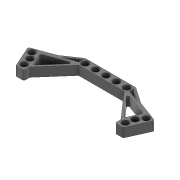
# Autodesk Inventor part: 2020-04-02-10-10501-LED_Splitter_Transparent
Saved by Autodesk Inventor 2020 (Build 240168000, 168)
## iProperties
Created: 2020-11-03
Part Number: 2020-04-02-10-10501-LED_Splitter_Transparent
Material: ABS Plastic
Document SubType Name: Modeling
Designer: eunde
Density: 1.06 g/cm^3
Appearance: Smooth - Black
Author: eunde
Autodesk Inventor part; units mm, degrees
ref_plane "YZ Plane" through (0, 0, 0) normal (1, 0, 0) x (0, 1, 0)
ref_plane "XZ Plane" through (0, 0, 0) normal (0, 1, 0) x (-1, 0, 0)
ref_plane "XY Plane" through (0, 0, 0) normal (0, 0, 1) x (1, 0, 0)
sketch "Sketch1" plane through (0, 0, 0) normal (0, 1, 0) x (-1, 0, 0)
  circle A0 centre (39, -6.055) radius 2.6
  circle A1 centre (40.5, -12.055) radius 2.6
  circle A2 centre (44, -17.055) radius 2.6
  line L0 (48.784, -18.8092) -> (41.3, -2)
  line L1 (0, 0) -> (60.8895, 0) construction
  line L2 (41.3, -2) -> (35.1, -2)
  circle A3 centre (16, -30.05) radius 2.6
  circle A4 centre (8, -30.05) radius 2.6
  arc A5 (0, -32.65) -> (0, -27.45) centre (0, -30.05) ccw
  line L3 (0, -33.55) -> (0, -32.65)
  line L4 (0, -27.45) -> (0, -26.55)
  line L5 (35.1, -2) -> (35.1, -6.5)
  line L6 (35.1, -8.7741) -> (39.6892, -19.0815)
  line L7 (0, -33.55) -> (19.5, -33.55)
  line L8 (19.5, -31.7318) -> (19.5, -28.6602)
  line L9 (19.5, -33.55) -> (31.902, -25.0543)
  line L10 (19.5, -31.7318) -> (29.2478, -25.0543)
  line L11 (17.5043, -26.55) -> (35.1, -6.5)
  line L12 (19.5, -26.55) -> (35.1, -8.7741)
  line L13 (19.5, -28.6602) -> (29.2478, -25.0543)
  line L14 (0, -26.55) -> (17.5043, -26.55)
  line L15 (39.6892, -19.0815) -> (19.5, -26.55)
  line L16 (48.784, -18.8092) -> (31.902, -25.0543)
  dimension "d0" = 5.2
  dimension "d1" = 1.5
  dimension "d3" = 3.5
  dimension "d5" = 6
  dimension "d6" = 5
  dimension "d12" = 39
  dimension "d14" = 114
  dimension "d15" = 18.4
  dimension "d16" = 6.055
  dimension "d17" = 6.2
  dimension "d19" = 30.05
  dimension "d21" = 8
  dimension "d22" = 5.2
  dimension "d26" = 3.9
  dimension "d29" = 19.5
  dimension "d31" = 18
  dimension "d35" = 1.5
  dimension "d37" = 1.5
  dimension "d40" = 3.5
  dimension "d41" = 3.5
  dimension "d44" = 4.5
  dimension "d45" = 0
  dimension "d46" = 8
  dimension "d48" = 2.9
  dimension "d49" = 2
  dimension "d51" = 0
  constraints: 34 end point, 7 vertical alignment, 6 centre point, 4 equal radius, 4 horizontal alignment, 3 horizontal, 3 vertical, 2 perpendicular, 2 point on circle
  measures "d0" diameter of A2
  measures "d1" horizontal distance of A0.centre A1.centre
  measures "d3" horizontal distance of A1.centre A2.centre
  measures "d5" vertical distance of A1.centre A0.centre
  measures "d6" vertical distance of A2.centre A1.centre
  measures "d12" horizontal distance of L1.start A0.centre
  measures "d14" angle of L1 L0
  measures "d15" distance of L0.start L0.end
  measures "d16" distance from line of L1 A0.centre
  measures "d17" distance of L0.end L2.end
  measures "d19" distance from line of L1 A3.centre
  measures "d21" distance of A3.centre A4.centre
  measures "d22" diameter of A5
  measures "d26" horizontal distance of L2.end A0.centre
  measures "d29" distance of L3.start L7.end
  measures "d31" distance of L9.end L0.start
  measures "d35" distance between parallel lines of L9 L10
  measures "d37" distance between parallel lines of L12 L11
  measures "d40" vertical distance of L3.start A4.centre
  measures "d41" distance of A5.centre L4.end
  measures "d44" distance of L2.end L5.end
  measures "d45" angle of L0 L6
  measures "d46" distance of A5.centre A4.centre
  measures "d48" distance between parallel lines of L16 L15
  measures "d49" distance between parallel lines of L1 L2
  measures "d51" angle of L13 L15
extrude "Extrusion1" add sketch "Sketch1" along normal blind 7
mirror "Mirror1" about plane through (0, 0, -32.65) normal (1, 0, 0) of "Extrusion1"
fillet "Fillet1" radius 1 18 edges at (-35.1, 3.5, -8.7741) (-39.6892, 3.5, -19.0815) (-19.5, 3.5, -26.55) (19.5, 3.5, -26.55) (39.6892, 3.5, -19.0815) (35.1, 3.5, -8.7741) (48.784, 3.5, -18.8092) (41.3, 3.5, -2) (35.1, 3.5, -2) (35.1, 3.5, -6.5) (-17.5043, 3.5, -26.55) (-35.1, 3.5, -6.5) (-35.1, 3.5, -2) (-41.3, 3.5, -2) (-48.784, 3.5, -18.8092) (-31.902, 3.5, -25.0543) (-19.5, 3.5, -33.55) (31.902, 3.5, -25.0543)
equation "\"d37\" = d34"
equation "\"d41\" = d40"
equation "\"d46\" = d21"
equation "\"d34\" = d35"
body "Solid1"
